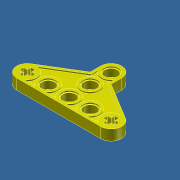
# Autodesk Inventor part: LEGO Brick 32017
Saved by Autodesk Inventor 2011 SP2 (Build 150553200, 553)
## iProperties
Company: Allseas Engineering BV
Created: 2011-11-29
Part Number: LEGO Brick 32017
Cost Center: 0 kg
Material: Steel
Document SubType Name: Modeling
Designer: BvH
Authority: 0 mm^3
Stock Number: =<Filenr>_<Document number>
Density: 7.85 g/cm^3
Mass: 11.459 g
Surface Area: 18.8328 cm^2
Volume: 1.45974 cm^3
Act. Code: DW000
SaveDate: 2011-07-28
SaveTime: 18:32
FileName: Standard
TotalMass: 0 kg
TotalVolume: 0 mm^3
Subject: =<Title><TITLE 1_2> <TITLE 2_2>
Author: BvH
Autodesk Inventor part; units mm, degrees
ref_plane "YZ Plane" through (0, 0, 0) normal (1, 0, 0) x (0, 1, 0)
ref_plane "XZ Plane" through (0, 0, 0) normal (0, 1, 0) x (-1, 0, 0)
ref_plane "XY Plane" through (0, 0, 0) normal (0, 0, 1) x (1, 0, 0)
sketch "Sketch1" plane through (0, 0, 0) normal (0, 0, 1) x (1, 0, 0)
  line L0 (0, -9.7468) -> (0, 24.9578) construction
  line L1 (-29.249, 0) -> (29.249, 0) construction
  arc A0 (-18.0821, 3.4154) -> (-16, -4) centre (-16, 0) ccw
  line L2 (-16, -4) -> (16, -4)
  arc A1 (16, -4) -> (18.0821, 3.4154) centre (16, 0) ccw
  line L3 (-18.0821, 3.4154) -> (-4, 12)
  line L4 (-4, 12) -> (-4, 16)
  arc A2 (4, 16) -> (-4, 16) centre (0, 16) ccw
  line L5 (4, 16) -> (4, 12)
  line L6 (4, 12) -> (18.0821, 3.4154)
  point P0 (0, -4)
  dimension "d0" = 40
  dimension "d38" = 8
  dimension "d39" = 24
  dimension "d41" = 4
  constraints: 10 end point, 6 point on circle, 6 tangent, 4 point on line, 3 centre point, 2 vertical, 1 equal radius, 1 horizontal, 1 midpoint, 1 parallel
  measures "d38" distance between parallel lines of L5 L4
  measures "d41" horizontal distance of A2.centre L5.end
sketch "Sketch8" plane through (0, 0, 0) normal (0, 0, 1) x (1, 0, 0)
  circle A0 centre (0, 0) radius 2.4
  circle A1 centre (0, 0) radius 2.75
  circle A2 centre (0, 16) radius 2.4
  circle A3 centre (0, 16) radius 2.75
  arc A4 (4, 16) -> (-4, 16) centre (0, 16) ccw construction
  line L0 (0, 16) -> (0, 0) construction
  circle A5 centre (0, 8) radius 2.4
  circle A6 centre (0, 8) radius 2.75
  circle A7 centre (-8, 0) radius 2.4
  circle A8 centre (-8, 0) radius 2.75
  circle A9 centre (8, 0) radius 2.4
  circle A10 centre (8, 0) radius 2.75
  line L1 (-8, 0) -> (8, 0) construction
  dimension "d42" = 5.5
  dimension "d43" = 4.8
  constraints: 10 centre point, 9 coincident, 8 equal radius, 4 end point, 2 midpoint, 1 horizontal, 1 perpendicular, 1 vertical
  measures "d42" diameter of A1
  measures "d43" diameter of A0
sketch "Sketch6" plane through (0, 0, 0) normal (0, 0, 1) x (1, 0, 0)
  arc A0 (-18.0821, 3.4154) -> (-16, -4) centre (-16, 0) ccw construction
  arc A1 (16, -4) -> (18.0821, 3.4154) centre (16, 0) ccw construction
  circle A2 centre (-16, 0) radius 2.3
  circle A3 centre (16, 0) radius 2.3
  line L0 (-18.1564, 0.8) -> (-16.8, 0.8)
  line L1 (-16.8, 0.8) -> (-16.8, 2.1564)
  line L2 (-15.2, 2.1564) -> (-15.2, 0.8)
  line L3 (-15.2, 0.8) -> (-13.8436, 0.8)
  line L4 (-13.8436, -0.8) -> (-15.2, -0.8)
  line L5 (-15.2, -0.8) -> (-15.2, -2.1564)
  line L6 (-16.8, -2.1564) -> (-16.8, -0.8)
  line L7 (-16.8, -0.8) -> (-18.1564, -0.8)
  line L8 (13.8436, 0.8) -> (15.2, 0.8)
  line L9 (16.8, 0.8) -> (18.1564, 0.8)
  line L10 (16.8, 2.1564) -> (16.8, 0.8)
  line L11 (16.8, -0.8) -> (16.8, -2.1564)
  line L12 (15.2, 2.1564) -> (15.2, 0.8)
  line L13 (15.2, -0.8) -> (15.2, -2.1564)
  line L14 (18.1564, -0.8) -> (16.8, -0.8)
  line L15 (15.2, -0.8) -> (13.8436, -0.8)
  circle A4 centre (-16, 0) radius 2.75
  circle A5 centre (16, 0) radius 2.75
  dimension "d29" = 4.6
  dimension "d30" = 1.6
  dimension "d44" = 5.5
  constraints: 32 end point, 13 equal length, 8 horizontal, 8 vertical, 4 coincident, 2 centre point, 2 collinear, 1 equal radius, 20 other
  measures "d30" distance between parallel lines of L2 L1
  measures "d44" diameter of A4
extrude "Extrusion1" add sketch "Sketch1" along normal mid plane 4
extrude "Extrusion9" cut sketch "Sketch6" along normal through all both and the other way through all contours A2 L4 L5 L6 L7 L0 L1 L2 L3 | A3 L14 L11 L13 L15 L8 L12 L10 L9
extrude "Extrusion10" cut sketch "Sketch8" along normal through all both and the other way through all contours A0 | A2 | A5 | A7 | A9
sketch "Sketch2" plane through (0, 0, 2) normal (0, 0, 1) x (1, 0, 0)
  circle A0 centre (0, 0) radius 2.75 projected
  circle A1 centre (-8, 0) radius 2.75 projected
  circle A2 centre (0, 8) radius 2.75 projected
  circle A3 centre (8, 0) radius 2.75 projected
  circle A4 centre (0, 16) radius 2.75 projected
extrude "Extrusion3" cut sketch "Sketch2" against normal blind 0.5333
sketch "Sketch3" plane through (0, 0, -2) normal (0, 0, -1) x (-1, 0, 0)
  circle A0 centre (0, 0) radius 2.75 projected
  circle A1 centre (-8, 0) radius 2.75 projected
  circle A2 centre (8, 0) radius 2.75 projected
  circle A3 centre (0, 8) radius 2.75 projected
  circle A4 centre (0, 16) radius 2.75 projected
extrude "Extrusion4" cut sketch "Sketch3" against normal blind 0.5333
sketch "Sketch9" plane through (0, 0, 2) normal (0, 0, 1) x (1, 0, 0)
  circle A0 centre (0, 16) radius 2.75 construction
  circle A1 centre (0, 8) radius 2.75 construction
  line L0 (4, 12) -> (18.0821, 3.4154) construction
  line L1 (-18.0821, 3.4154) -> (-4, 12) construction
  circle A2 centre (-8, 0) radius 2.75 construction
  circle A3 centre (0, 0) radius 2.75 construction
  circle A4 centre (8, 0) radius 2.75 construction
  circle A5 centre (-16, 0) radius 2.75 construction
  circle A6 centre (16, 0) radius 2.75 construction
  line L2 (1.3037, 12.6027) -> (16.0078, 3.6389)
  arc A7 (16.0078, 3.6389) -> (14.1125, -3.1111) centre (16, 0) ccw
  line L3 (-16.0078, 3.6389) -> (-1.3037, 12.6027)
  arc A8 (-14.1125, -3.1111) -> (-16.0078, 3.6389) centre (-16, 0) ccw
  line L4 (-28, 0) -> (28, 0) construction
  line L5 (0, -8.8) -> (0, 24.8) construction
  line L6 (16, -4) -> (-16, -4) construction
  arc A9 (-6.1125, -3.1111) -> (-9.8875, -3.1111) centre (-8, 0) ccw
  line L7 (-14.1125, -3.1111) -> (-9.8875, -3.1111)
  line L8 (-6.1125, -3.1111) -> (-1.8875, -3.1111)
  arc A10 (1.8875, -3.1111) -> (-1.8875, -3.1111) centre (0, 0) ccw
  line L9 (1.8875, -3.1111) -> (6.1125, -3.1111)
  arc A11 (9.8875, -3.1111) -> (6.1125, -3.1111) centre (8, 0) ccw
  line L10 (9.8875, -3.1111) -> (14.1125, -3.1111)
  arc A12 (-3.1111, 14.1125) -> (3.1111, 14.1125) centre (0, 16) ccw
  arc A13 (3.1111, 9.8875) -> (-3.1111, 9.8875) centre (0, 8) ccw
  line L11 (-3.1111, 14.1125) -> (-3.1111, 9.8875)
  line L12 (3.1111, 14.1125) -> (3.1111, 9.8875)
  line L13 (-4, 12) -> (-4, 16) construction
  line L14 (4, 16) -> (4, 12) construction
  arc A14 (-0.6774, 11.5753) -> (0.6774, 11.5753) centre (0, 8) ccw
  line L15 (1.3037, 12.6027) -> (0.6774, 11.5753)
  line L16 (-1.3037, 12.6027) -> (-0.6774, 11.5753)
  dimension "d52" = 0.8889
  dimension "d53" = 0.8889
  dimension "d54" = 0.8889
  dimension "d55" = 0.8889
  dimension "d58" = 0.8889
  dimension "d59" = 0.8889
  constraints: 20 end point, 18 point on circle, 8 centre point, 8 coincident, 7 equal radius, 4 horizontal, 3 collinear, 2 parallel, 2 perpendicular, 2 vertical
  measures "d52" radial gap between concentric circles of A7 A6
  measures "d53" distance between parallel lines of L0 L2
  measures "d54" distance between parallel lines of L1 L3
  measures "d55" distance between parallel lines of L6 L7
  measures "d58" distance between parallel lines of L14 L12
  measures "d59" distance between parallel lines of L13 L11
extrude "Extrusion11" cut sketch "Sketch9" against normal blind 0.5333 contours A12 L12 L2 | L15 A13 L16 A12 | L2 L12 A13 L15 | L2 A7 L10 A11 L9 A10 L8 A9 L7 A8 L3 L11 A14 L12 | L16 A13 L11 L3 | L3 L11 A12
sketch "Sketch10" plane through (0, 0, -2) normal (0, 0, -1) x (-1, 0, 0)
  arc A0 (-3.1111, 14.1125) -> (3.1111, 14.1125) centre (0, 16) ccw projected
  line L0 (3.1111, 14.1125) -> (3.1111, 11.5008) projected
  line L1 (3.1111, 11.5008) -> (16.0078, 3.6389) projected
  arc A1 (16.0078, 3.6389) -> (14.1125, -3.1111) centre (16, 0) ccw projected
  line L2 (14.1125, -3.1111) -> (9.8875, -3.1111) projected
  arc A2 (9.8875, -3.1111) -> (6.1125, -3.1111) centre (8, 0) ccw projected
  line L3 (6.1125, -3.1111) -> (1.8875, -3.1111) projected
  arc A3 (1.8875, -3.1111) -> (-1.8875, -3.1111) centre (0, 0) ccw projected
  line L4 (-1.8875, -3.1111) -> (-6.1125, -3.1111) projected
  arc A4 (-6.1125, -3.1111) -> (-9.8875, -3.1111) centre (-8, 0) ccw projected
  line L5 (-9.8875, -3.1111) -> (-14.1125, -3.1111) projected
  arc A5 (-14.1125, -3.1111) -> (-16.0078, 3.6389) centre (-16, 0) ccw projected
  line L6 (-16.0078, 3.6389) -> (-3.1111, 11.5008) projected
  line L7 (-3.1111, 11.5008) -> (-3.1111, 14.1125) projected
  circle A6 centre (0, 8) radius 3.6389 projected
extrude "Extrusion12" cut sketch "Sketch10" against normal blind 0.5333
equation "\"d38\" = width_standard"
equation "\"d41\" = 0.5 * width_standard"
equation "\"d2\" = 0.5 * width_standard"
equation "\"d13\" = 0.0555556 * height_standard"
equation "\"d15\" = 0.0555556 * height_standard"
equation "\"d56\" = 0.0555556 * height_standard"
equation "\"d60\" = 0.0555556 * height_standard"
equation "\"width_standard\" = 8"
equation "\"height_standard\" = 9.6"
body "Solid1"
